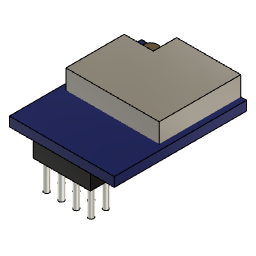
MLH4 v1.0 (Autodesk Fusion 360 archive; units mm, degrees)
design "RA-02"
Autodesk Fusion 360 part; units mm, degrees
sketch "Esquisse1" plane through (0, 0, 0) normal (0, 0, 1) x (1, 0, 0) in component "LoRa RA-02"
  line L0 (0, 0) -> (18, 0)
  line L1 (18, 0) -> (18, -22.7)
  line L2 (18, -22.7) -> (0, -22.7)
  line L3 (0, -22.7) -> (0, 0)
  line L4 (1, 0) -> (17, 0)
  line L5 (17, 0) -> (17, -14)
  line L6 (17, -14) -> (1, -14)
  line L7 (1, -14) -> (1, 0)
  line L8 (13.9, -22.7) -> (4.1, -22.7)
  line L9 (4.1, -22.7) -> (4.1, -17.7)
  line L10 (4.1, -17.7) -> (13.9, -17.7)
  line L11 (13.9, -17.7) -> (13.9, -22.7)
  line L12 (1, 0) -> (6, 0)
  line L13 (6, 0) -> (6, -4)
  line L14 (6, -4) -> (1, -4)
  line L15 (1, -4) -> (1, 0)
  circle A0 centre (3.5142, -2) radius 1.25
  circle A1 centre (5.2, -21.5) radius 0.445
  circle A2 centre (7.74, -21.5) radius 0.445
  circle A3 centre (10.28, -21.5) radius 0.445
  circle A4 centre (12.82, -21.5) radius 0.445
  circle A5 centre (5.2, -18.96) radius 0.445
  circle A6 centre (7.74, -18.96) radius 0.445
  circle A7 centre (10.28, -18.96) radius 0.445
  circle A8 centre (12.82, -18.96) radius 0.445
  dimension "d1" = 18
  dimension "d2" = 22.7
  dimension "d3" = 16
  dimension "d4" = 14
  dimension "d5" = 9.8
  dimension "d6" = 5
  dimension "d7" = 5
  dimension "d8" = 4
  dimension "d9" = 2.5
  dimension "d18" = 0.89
  dimension "d21" = 7.62
  dimension "d22" = 2.54
  dimension "d23" = 1.2
  dimension "d24" = 1.1
  constraint horizontal L0
  constraint vertical L1
  constraint horizontal L2
  constraint vertical L3
  constraint coincident L0.start L3.end
  constraint horizontal L4
  constraint vertical L5
  constraint horizontal L6
  constraint vertical L7
  constraint coincident L0 L4.start
  constraint midpoint L0 L4
  constraint horizontal L8
  constraint vertical L9
  constraint horizontal L10
  constraint vertical L11
  constraint coincident L2 L8.start
  constraint midpoint L2 L8
  constraint horizontal L12
  constraint vertical L13
  constraint horizontal L14
  constraint vertical L15
  measures "d1" distance of L0.start L0.end
  measures "d2" distance of L0.start L2.end
  measures "d3" distance of L4.start L4.end
  measures "d4" distance of L4.start L6.end
  measures "d5" distance of L8.start L8.end
  measures "d6" distance of L8.start L10.end
  measures "d7" distance of L4.start L12.end
  measures "d8" distance of L4.start L14.end
  measures "d9" diameter of A0
  measures "d18" diameter of A1
  measures "d23" distance of L2 A1.centre
  measures "d24" distance of L9 A1.centre
extrude "Extrusion1" add sketch "Esquisse1" along normal blind 1.6 contours L0 L1 L2 L3 L5 L6 L7 L9 L10 L11 L15 | L0 L4 L7 L12 L13 L14 L15 | L0 L4 L5 L6 L7 L13 L14 | L2 L8 L9 L10 L11 | A0 | A1 | A2 | A3 | A4 | A5 | A6 | A7 | A8 makes body 1 in component "LoRa RA-02"
extrude "Extrusion2" add sketch "Esquisse1" against normal blind 2.6 separate body contours L2 L8 L9 L10 L11 | A1 | A2 | A3 | A4 | A5 | A6 | A7 | A8 makes body 2 in component "LoRa RA-02"
extrude "Extrusion3" add sketch "Esquisse1" along normal blind 4.9 separate body contours L0 L4 L5 L6 L7 L13 L14 makes body 3 in component "LoRa RA-02"
extrude "Extrusion4" add sketch "Esquisse1" along normal blind 3 separate body contours A0 makes body 4 in component "LoRa RA-02"
extrude "Extrusion5" add sketch "Esquisse1" against normal blind 5 from surface at -2.6 separate body contours A1 | A2 | A3 | A4 | A5 | A6 | A7 | A8 makes body 5 at (10.077, -19.356, -4.2667) makes body 6 at (8.1712, -21.6098, -5.9333) makes body 7 at (12.617, -21.896, -4.2667) makes body 8 at (8.1712, -19.0698, -5.9333) makes body 9 at (12.617, -19.356, -4.2667) makes body 10 at (5.6312, -21.6098, -5.9333) makes body 11 at (10.077, -21.896, -4.2667) makes body 12 at (5.6312, -19.0698, -5.9333) in component "LoRa RA-02"
component "LoRa RA-02" placed x (1, 0, 0) y (0, 1, 0) z (0, 0, 1) at (0, 0, 0)
named bodies: "PCB", "connecteur", "SX11278", "IPX"

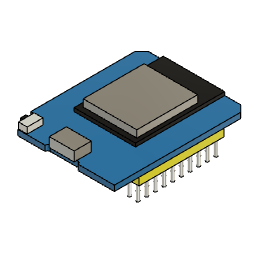
design "D1-mini32"
Autodesk Fusion 360 part; units mm, degrees
sketch "Esquisse1" plane through (0, 0, 0) normal (0, 0, 1) x (1, 0, 0) in component "D1-MINI-32"
  line L0 (15.6, -19.8) -> (-15.4, -19.8)
  line L1 (-15.4, -19.8) -> (-15.4, 19.2)
  line L2 (-15.4, 19.2) -> (15.6, 19.2)
  line L3 (15.6, 19.2) -> (15.6, -19.8)
  line L4 (15.4, 12.6) -> (10.4, 12.6)
  line L5 (10.4, 12.6) -> (10.4, -12.4)
  line L6 (10.4, -12.4) -> (15.4, -12.4)
  line L7 (15.4, -12.4) -> (15.4, 12.6)
  line L8 (-15.2, -12.4) -> (-10.2, -12.4)
  line L9 (-10.2, -12.4) -> (-10.2, 12.6)
  line L10 (-10.2, 12.6) -> (-15.2, 12.6)
  line L11 (-15.2, 12.6) -> (-15.2, -12.4)
  circle A0 centre (-13.85, -14.45) radius 1.0794
  line L12 (-13.85, -13.3706) -> (-15.4, -13.3707)
  line L13 (-12.7712, -14.4847) -> (-12.7712, -19.8)
  line L14 (-15.4, 17.2481) -> (-13.3669, 19.2)
  line L15 (15.6, 17.2735) -> (13.7505, 19.2)
  circle A1 centre (-4, -19.8) radius 0.7616
  circle A2 centre (4.2, -19.8) radius 0.76
  line L16 (-4.0175, -19.0386) -> (4.2001, -19.04)
  circle A3 centre (-13.87, 11.56) radius 0.4445
  circle A4 centre (-11.33, 11.56) radius 0.4445
  circle A5 centre (-13.87, 9.02) radius 0.4445
  circle A6 centre (-11.33, 9.02) radius 0.4445
  circle A7 centre (-13.87, 6.48) radius 0.4445
  circle A8 centre (-11.33, 6.48) radius 0.4445
  circle A9 centre (-13.87, 3.94) radius 0.4445
  circle A10 centre (-11.33, 3.94) radius 0.4445
  circle A11 centre (-13.87, 1.4) radius 0.4445
  circle A12 centre (-11.33, 1.4) radius 0.4445
  circle A13 centre (-13.87, -1.14) radius 0.4445
  circle A14 centre (-11.33, -1.14) radius 0.4445
  circle A15 centre (-13.87, -3.68) radius 0.4445
  circle A16 centre (-11.33, -3.68) radius 0.4445
  circle A17 centre (-13.87, -6.22) radius 0.4445
  circle A18 centre (-11.33, -6.22) radius 0.4445
  circle A19 centre (-13.87, -8.76) radius 0.4445
  circle A20 centre (-11.33, -8.76) radius 0.4445
  circle A21 centre (-13.87, -11.3) radius 0.4445
  circle A22 centre (-11.33, -11.3) radius 0.4445
  circle A23 centre (11.53, 11.56) radius 0.4445
  circle A24 centre (14.07, 11.56) radius 0.4445
  circle A25 centre (11.53, 9.02) radius 0.4445
  circle A26 centre (14.07, 9.02) radius 0.4445
  circle A27 centre (11.53, 6.48) radius 0.4445
  circle A28 centre (14.07, 6.48) radius 0.4445
  circle A29 centre (11.53, 3.94) radius 0.4445
  circle A30 centre (14.07, 3.94) radius 0.4445
  circle A31 centre (11.53, 1.4) radius 0.4445
  circle A32 centre (14.07, 1.4) radius 0.4445
  circle A33 centre (11.53, -1.14) radius 0.4445
  circle A34 centre (14.07, -1.14) radius 0.4445
  circle A35 centre (11.53, -3.68) radius 0.4445
  circle A36 centre (14.07, -3.68) radius 0.4445
  circle A37 centre (11.53, -6.22) radius 0.4445
  circle A38 centre (14.07, -6.22) radius 0.4445
  circle A39 centre (11.53, -8.76) radius 0.4445
  circle A40 centre (14.07, -8.76) radius 0.4445
  circle A41 centre (11.53, -11.3) radius 0.4445
  circle A42 centre (14.07, -11.3) radius 0.4445
  dimension "d1" = 31
  dimension "d2" = 39
  dimension "d3" = 5
  dimension "d4" = 25
  dimension "d5" = 5
  dimension "d6" = 25
  dimension "d22" = 1.52
  dimension "d23" = 0.889
  dimension "d28" = 2.54
  dimension "d29" = -22.86
  dimension "d30" = 8.5
  dimension "d31" = 0.889
  dimension "d32" = 25.4
  dimension "d35" = 2.54
  dimension "d36" = -22.86
  dimension "d37" = 8.5
  dimension "d39" = 1.53
  constraint horizontal L0
  constraint vertical L1
  constraint horizontal L2
  constraint vertical L3
  constraint horizontal L4
  constraint vertical L5
  constraint horizontal L6
  constraint vertical L7
  constraint horizontal L8
  constraint vertical L9
  constraint horizontal L10
  constraint vertical L11
  constraint coincident A0 L12.start
  constraint coincident L1 L12.end
  constraint tangent A0 L12
  constraint coincident A0 L13.start
  constraint coincident L0 L13.end
  constraint perpendicular L0 L13
  constraint coincident L1 L14.start
  constraint coincident L2 L14.end
  constraint coincident L3 L15.start
  constraint coincident L2 L15.end
  constraint perpendicular L14 L15
  constraint coincident L0 A1.centre
  constraint coincident L0 A2.centre
  constraint coincident A1 L16.start
  constraint coincident A2 L16.end
  constraint tangent A2 L16
  measures "d1" distance of L0.start L0.end
  measures "d2" distance of L0.start L2.end
  measures "d3" distance of L4.start L4.end
  measures "d4" distance of L4.start L6.end
  measures "d5" distance of L8.start L8.end
  measures "d6" distance of L8.start L10.end
  measures "d22" diameter of A2
  measures "d23" diameter of A3
  measures "d30" distance of L0 A21.centre
  measures "d31" diameter of A23
  measures "d32" horizontal distance of A3.centre A23.centre
  measures "d37" distance of L0 A41.centre
  measures "d39" distance of L1 A3.centre
extrude "Extrusion1" add sketch "Esquisse1" along normal blind 1.6 contours L0 L1 L2 L3 A0 L12 L13 L14 L15 A1 A2 L16 | L4 L5 L6 L7 | L8 L9 L10 L11 | A3 | A4 | A5 | A6 | A7 | A8 | A9 | A10 | A11 | A12 | A13 | A14 | A15 | A16 | A17 | A18 | A19 | A20 | A21 | A22 | A23 | A24 | A25 | A26 | A27 | A28 | A29 | A30 | A31 | A32 | A33 | A34 | A35 | A36 | A37 | A38 | A39 | A40 | A41 | A42 makes body 1 in component "D1-MINI-32"
extrude "Extrusion2" add sketch "Esquisse1" against normal blind 2.4 separate body contours L4 L5 L6 L7 | L8 L9 L10 L11 | A3 | A4 | A5 | A6 | A7 | A8 | A9 | A10 | A11 | A12 | A13 | A14 | A15 | A16 | A17 | A18 | A19 | A20 | A21 | A22 | A23 | A24 | A25 | A26 | A27 | A28 | A29 | A30 | A31 | A32 | A33 | A34 | A35 | A36 | A37 | A38 | A39 | A40 | A41 | A42 makes body 2 at (-13.5333, 4.2667, 0) makes body 3 at (12.0667, 4.2667, 0) in component "D1-MINI-32"
sketch "Esquisse2" plane through (0, 0, 1.6) normal (0, 0, 1) x (-1, 0, 0) in component "D1-MINI-32"
  line L0 (-13.7505, -19.2) -> (13.3669, -19.2)
  line L1 (15.4, -17.2481) -> (15.4, 13.3707)
  line L2 (-4.96, 19.8) -> (-15.6, 19.8)
  line L3 (-15.6, 19.8) -> (-15.6, -17.2735)
  line L4 (3.507, 19.8) -> (-3.7943, 19.8)
  line L5 (-3.7943, 19.8) -> (-3.7943, 14.7793)
  line L6 (-3.7943, 14.7793) -> (3.507, 14.7793)
  line L7 (3.507, 14.7793) -> (3.507, 19.8)
  line L8 (9.0381, -19.2) -> (-9, -19.2)
  line L9 (-9, -19.2) -> (-9, 7)
  line L10 (-9, 7) -> (9.0381, 7)
  line L11 (9.0381, 7) -> (9.0381, -19.2)
  line L12 (7.8495, -12.3669) -> (-7.9109, -12.3669)
  line L13 (-7.9109, -12.3669) -> (-7.9109, 5.5066)
  line L14 (-7.9109, 5.5066) -> (7.8495, 5.5066)
  line L15 (7.8495, 5.5066) -> (7.8495, -12.3669)
  arc A0 (12.7712, 14.4847) -> (13.85, 13.3706) centre (13.85, 14.45) ccw
  line L16 (12.7712, 14.4847) -> (12.7712, 19.8)
  line L17 (15.4, 13.3707) -> (13.85, 13.3706)
  line L18 (10.2, 19.6) -> (12.7712, 19.6)
  line L19 (12.7712, 19.6) -> (12.7712, 14.9726)
  line L20 (12.7712, 14.9726) -> (10.2, 14.9726)
  line L21 (10.2, 14.9726) -> (10.2, 19.6)
  line L22 (12.7712, 16.4284) -> (13.7, 16.4284)
  line L23 (13.7, 16.4284) -> (13.7, 18.1)
  line L24 (13.7, 18.1) -> (12.7712, 18.1)
  line L25 (12.7712, 18.1) -> (12.7712, 16.4284)
  arc A1 (4.0175, 19.0386) -> (4.7616, 19.8) centre (4, 19.8) ccw
  line L26 (4.0175, 19.0386) -> (-4.2001, 19.04)
  arc A2 (-4.96, 19.8) -> (-4.2001, 19.04) centre (-4.2, 19.8) ccw
  line L27 (-15.6, -17.2735) -> (-13.7505, -19.2)
  line L28 (13.3669, -19.2) -> (15.4, -17.2481)
  line L29 (12.7712, 19.8) -> (4.7616, 19.8)
  constraint horizontal L4
  constraint vertical L5
  constraint horizontal L6
  constraint vertical L7
  constraint coincident L2 L4.start
  constraint horizontal L8
  constraint vertical L9
  constraint horizontal L10
  constraint vertical L11
  constraint coincident L0 L8.start
  constraint horizontal L12
  constraint vertical L13
  constraint horizontal L14
  constraint vertical L15
  constraint horizontal L18
  constraint vertical L19
  constraint horizontal L20
  constraint vertical L21
  constraint coincident L16 L19.end
  constraint horizontal L22
  constraint vertical L23
  constraint horizontal L24
  constraint vertical L25
  constraint coincident L16 L22.start
extrude "Extrusion3" add sketch "Esquisse2" along normal blind 2.8 separate body contours L5 L6 L7 L26 | L4 L5 L7 L26 makes body 4 in component "D1-MINI-32"
extrude "Extrusion4" add sketch "Esquisse2" along normal blind 1 separate body contours L0 L8 L9 L10 L11 makes body 5 in component "D1-MINI-32"
extrude "Extrusion5" add sketch "Esquisse2" along normal blind 3.1 separate body contours L12 L13 L14 L15 makes body 6 in component "D1-MINI-32"
extrude "Extrusion6" add sketch "Esquisse2" along normal blind 1.8 separate body contours L16 L18 L19 L20 L21 L25 makes body 7 in component "D1-MINI-32"
extrude "Extrusion7" add sketch "Esquisse2" along normal blind 1.4 from surface at 0.2 separate body contours L16 L19 L22 L23 L24 L25 makes body 8 in component "D1-MINI-32"
extrude "Extrusion8" add sketch "Esquisse1" against normal blind 5 from surface at -2.4 separate body contours A3 | A4 | A5 | A6 | A7 | A8 | A9 | A10 | A11 | A12 | A13 | A14 | A15 | A16 | A17 | A18 | A19 | A20 | A21 | A22 | A23 | A24 | A25 | A26 | A27 | A28 | A29 | A30 | A31 | A32 | A33 | A34 | A35 | A36 | A37 | A38 | A39 | A40 | A41 | A42 makes body 9 at (-11.2096, -8.3321, -5.7333) makes body 10 at (-13.7496, -3.2521, -5.7333) makes body 11 at (-13.7496, 1.8279, -5.7333) makes body 12 at (-11.2096, 6.9079, -5.7333) makes body 13 at (-11.2096, 11.9879, -5.7333) makes body 14 at (11.7712, 6.8534, -5.7333) makes body 15 at (14.4796, 4.1127, -5.7333) makes body 16 at (11.7712, -0.7666, -5.7333) makes body 17 at (11.9396, -6.0473, -5.7333) makes body 18 at (11.1507, -11.0682, -5.7333) makes body 19 at (11.7712, -8.3866, -5.7333) makes body 20 at (11.9739, -3.7022, -5.7333) makes body 21 at (14.3112, 11.9334, -5.7333) makes body 22 at (14.3112, 1.7734, -5.7333) makes body 23 at (11.1507, 9.2518, -5.7333) makes body 24 at (-11.2096, 9.4479, -5.7333) makes body 25 at (-11.2096, 4.3679, -5.7333) makes body 26 at (-11.2096, -0.7121, -5.7333) makes body 27 at (-11.2096, -5.7921, -5.7333) makes body 28 at (-11.2096, -10.8721, -5.7333) makes body 29 at (-13.7496, -8.3321, -5.7333) makes body 30 at (-11.2096, -3.2521, -5.7333) makes body 31 at (-11.2096, 1.8279, -5.7333) makes body 32 at (-13.7496, 6.9079, -5.7333) makes body 33 at (-13.7496, 11.9879, -5.7333) makes body 34 at (11.9396, 4.1127, -5.7333) makes body 35 at (14.3112, 6.8534, -5.7333) makes body 36 at (14.3112, -0.7666, -5.7333) makes body 37 at (14.4796, -6.0473, -5.7333) makes body 38 at (13.6907, -11.0682, -5.7333) makes body 39 at (14.3112, -8.3866, -5.7333) makes body 40 at (14.5139, -3.7022, -5.7333) makes body 41 at (13.6907, 9.2518, -5.7333) makes body 42 at (11.7712, 1.7734, -5.7333) makes body 43 at (11.7712, 11.9334, -5.7333) makes body 44 at (-13.7496, 9.4479, -5.7333) makes body 45 at (-13.7496, 4.3679, -5.7333) makes body 46 at (-13.7496, -0.7121, -5.7333) makes body 47 at (-13.7496, -5.7921, -5.7333) makes body 48 at (-13.7496, -10.8721, -5.7333) in component "D1-MINI-32"
component "D1-MINI-32" placed x (1, 0, 0) y (0, 1, 0) z (0, 0, 1) at (0, 0, 0)
named bodies: "PCB", "J1", "J2", "USB", "Antenna", "ESP32 wroom", "inter", "bp"
